Autodesk Fusion 360 part; units mm, degrees
note: some values were not read from the file. Set by a fixed rule: which sketch regions a step uses.
(part 2 of 2)
  arc A362 (-112.6, 171.1932) -> (-113.4, 170.3932) centre (-112.6, 170.3932) ccw construction
  line L338 (-117.9, 167.3932) -> (-117.9, 156.3932)
  line L339 (-117.7203, 171.6851) -> (-116.5919, 172.8135)
  line L340 (-113.9, 169.6932) -> (-113.9, 158.6932)
  line L341 (-106.1426, 173.4432) -> (-115.0716, 173.4432)
  arc A363 (-132.4, 155.6932) -> (-131.6, 154.8932) centre (-131.6, 155.6932) ccw construction
  arc A364 (-111.9, 171.6932) -> (-113.9, 169.6932) centre (-111.9, 169.6932) ccw
  line L342 (-113.4, 170.3932) -> (-113.4, 157.9932) construction
  arc A365 (-131.6, 149.8932) -> (-132.4, 149.0932) centre (-131.6, 149.0932) ccw construction
  arc A366 (-132.9, 156.3932) -> (-130.9, 154.3932) centre (-130.9, 156.3932) ccw
  line L343 (-117.6142, 171.579) -> (-116.4858, 172.7074) construction
  circle A367 centre (-115.9, 153.5432) radius 1.5
  arc A368 (-117.9, 167.3932) -> (-119.9, 169.3932) centre (-119.9, 167.3932) ccw
  line L344 (-118.4, 168.0932) -> (-118.4, 155.6932) construction
  arc A369 (-94.4, 165.9932) -> (-93.6, 165.1932) centre (-93.6, 165.9932) ccw construction
  line L345 (-92.9, 160.6932) -> (-81.9, 160.6932)
  arc A370 (-93.6, 160.1932) -> (-94.4, 159.3932) centre (-93.6, 159.3932) ccw construction
  arc A371 (-100.2, 157.1932) -> (-99.4, 157.9932) centre (-100.2, 157.9932) ccw construction
  arc A372 (-79.9, 158.6932) -> (-81.9, 160.6932) centre (-81.9, 158.6932) ccw
  arc A373 (-81.2, 165.1932) -> (-80.4, 165.9932) centre (-81.2, 165.9932) ccw construction
  arc A374 (-74.6, 163.6932) -> (-75.4, 162.8932) centre (-74.6, 162.8932) ccw construction
  arc A375 (-100.9, 156.6932) -> (-98.9, 158.6932) centre (-100.9, 158.6932) ccw
  arc A376 (-92.9, 160.6932) -> (-94.9, 158.6932) centre (-92.9, 158.6932) ccw
  arc A377 (-94.9, 166.6932) -> (-92.9, 164.6932) centre (-92.9, 166.6932) ccw
  line L346 (-93.6, 165.1932) -> (-81.2, 165.1932) construction
  arc A378 (-73.9, 164.1932) -> (-75.9, 162.1932) centre (-73.9, 162.1932) ccw
  arc A379 (-80.4, 159.3932) -> (-81.2, 160.1932) centre (-81.2, 159.3932) ccw construction
  arc A380 (-81.9, 164.6932) -> (-79.9, 166.6932) centre (-81.9, 166.6932) ccw
  line L347 (-92.9, 164.6932) -> (-81.9, 164.6932)
  arc A381 (-82.2284, 181.4432) -> (-80.9203, 181.9851) centre (-82.2284, 183.2932) ccw
  arc A382 (-73.9, 183.1932) -> (-75.9, 181.1932) centre (-73.9, 181.1932) ccw
  line L348 (-93.6, 160.1932) -> (-81.2, 160.1932) construction
  arc A383 (-82.2284, 181.2932) -> (-80.8142, 181.879) centre (-82.2284, 183.2932) ccw construction
  arc A384 (-96.0716, 181.2932) -> (-97.4858, 180.7074) centre (-96.0716, 179.2933) ccw construction
  line L349 (-96.0716, 181.2932) -> (-82.2284, 181.2932) construction
  arc A385 (-93.6, 179.1932) -> (-94.4, 178.3932) centre (-93.6, 178.3932) ccw construction
  line L350 (-77.0716, 184.9432) -> (-59.7284, 184.9432)
  arc A386 (-92.9, 179.6932) -> (-94.9, 177.6932) centre (-92.9, 177.6932) ccw
  arc A387 (-96.0716, 181.4432) -> (-97.5918, 180.8135) centre (-96.0716, 179.2933) ccw
  line L351 (-78.4858, 184.2074) -> (-80.8142, 181.879) construction
  arc A388 (-77.0716, 184.7932) -> (-78.4858, 184.2074) centre (-77.0716, 182.7933) ccw construction
  arc A389 (-75.9, 170.1932) -> (-73.9, 168.1932) centre (-73.9, 170.1932) ccw
  line L352 (-92.9, 179.6932) -> (-81.9, 179.6932)
  line L353 (-96.0716, 181.4432) -> (-82.2284, 181.4432)
  arc A390 (-79.9, 177.6932) -> (-81.9, 179.6932) centre (-81.9, 177.6932) ccw
  line L354 (-94.9, 177.6932) -> (-94.9, 166.6932)
  line L355 (-94.4, 178.3932) -> (-94.4, 165.9932) construction
  line L356 (-73.9, 164.1932) -> (-62.9, 164.1932)
  line L357 (-79.9, 177.6932) -> (-79.9, 166.6932)
  arc A391 (-77.0716, 184.9432) -> (-78.5919, 184.3135) centre (-77.0716, 182.7933) ccw
  arc A392 (-75.4, 169.4932) -> (-74.6, 168.6932) centre (-74.6, 169.4932) ccw construction
  line L358 (-75.4, 181.8932) -> (-75.4, 169.4932) construction
  line L359 (-80.4, 178.3932) -> (-80.4, 165.9932) construction
  line L360 (-73.9, 183.1932) -> (-62.9, 183.1932)
  line L361 (-78.5919, 184.3135) -> (-80.9203, 181.9851)
  line L362 (-98.9, 169.6932) -> (-98.9, 158.6932)
  arc A393 (-98.9, 169.6932) -> (-100.9, 171.6932) centre (-100.9, 169.6932) ccw
  line L363 (-75.9, 181.1932) -> (-75.9, 170.1932)
  line L364 (-93.6, 179.1932) -> (-81.2, 179.1932) construction
  arc A394 (-80.4, 178.3932) -> (-81.2, 179.1932) centre (-81.2, 178.3932) ccw construction
  arc A395 (-74.6, 182.6932) -> (-75.4, 181.8932) centre (-74.6, 181.8932) ccw construction
  arc A396 (-99.4, 170.3932) -> (-100.2, 171.1932) centre (-100.2, 170.3932) ccw construction
  line L365 (-99.4, 170.3932) -> (-99.4, 157.9932) construction
  line L366 (-73.9, 168.1932) -> (-62.9, 168.1932)
  line L367 (-80.4, 159.3932) -> (-80.4, 146.9932) construction
  line L368 (-75.4, 162.8932) -> (-75.4, 150.4932) construction
  line L369 (-74.6, 144.6932) -> (-62.2, 144.6932) construction
  circle A397 centre (-63.3, 123.4932) radius 1.5 construction
  circle A398 centre (-63.3, 123.4932) radius 3.8
  line L370 (-74.6, 130.6932) -> (-62.2, 130.6932) construction
  line L371 (-94.4, 159.3932) -> (-94.4, 146.9932) construction
  line L372 (-73.9, 149.1932) -> (-62.9, 149.1932)
  line L373 (-74.6, 182.6932) -> (-62.2, 182.6932) construction
  line L374 (-75.9, 162.1932) -> (-75.9, 151.1932)
  line L375 (-74.6, 149.6932) -> (-62.2, 149.6932) construction
  line L376 (-94.9, 158.6932) -> (-94.9, 147.6932)
  line L377 (-59.6047, 106.0356) -> (-67.8823, 120.687)
  line L378 (-74.6, 163.6932) -> (-62.2, 163.6932) construction
  line L379 (-79.9, 158.6932) -> (-79.9, 147.6932)
  line L380 (-73.9, 130.1932) -> (-62.9, 130.1932)
  line L381 (-36.6, 118.8932) -> (-24.2, 118.8932) construction
  line L382 (-36.6, 137.8932) -> (-24.2, 137.8932) construction
  line L383 (-35.9, 138.3932) -> (-24.9, 138.3932)
  line L384 (-39.0716, 102.6432) -> (-24.0284, 102.6432)
  line L385 (-36.6, 123.8932) -> (-24.2, 123.8932) construction
  circle A399 centre (-39.9, 122.5432) radius 1.5
  line L386 (-35.9, 119.3932) -> (-24.9, 119.3932)
  line L387 (-36.6, 104.8932) -> (-24.2, 104.8932) construction
  line L388 (-39.0716, 102.7932) -> (-24.0284, 102.7932) construction
  line L389 (-43.0284, 105.0932) -> (-57.7328, 105.0932) construction
  line L390 (-35.9, 123.3932) -> (-24.9, 123.3932)
  line L391 (-35.9, 104.3932) -> (-24.9, 104.3932)
  arc A400 (-37.9, 125.3932) -> (-35.9, 123.3932) centre (-35.9, 125.3932) ccw
  line L392 (-55.6, 107.1932) -> (-43.2, 107.1932) construction
  arc A401 (-41.6142, 104.5074) -> (-43.0284, 105.0932) centre (-43.0284, 103.0933) ccw construction
  arc A402 (-37.4, 105.6932) -> (-36.6, 104.8932) centre (-36.6, 105.6932) ccw construction
  line L393 (-55.6, 121.1932) -> (-43.2, 121.1932) construction
  arc A403 (-56.4, 107.9932) -> (-55.6, 107.1932) centre (-55.6, 107.9932) ccw construction
  line L394 (-40.4858, 103.379) -> (-41.6142, 104.5074) construction
  arc A404 (-59.6047, 106.0356) -> (-57.7328, 104.9432) centre (-57.7328, 107.0932) ccw
  arc A405 (-35.9, 119.3932) -> (-37.9, 117.3932) centre (-35.9, 117.3932) ccw
  line L395 (-56.9, 119.6932) -> (-56.9, 108.6932)
  arc A406 (-54.9, 121.6932) -> (-56.9, 119.6932) centre (-54.9, 119.6932) ccw
  line L396 (-56.4, 120.3932) -> (-56.4, 107.9932) construction
  arc A407 (-41.7203, 104.4013) -> (-43.0284, 104.9432) centre (-43.0284, 103.0933) ccw
  arc A408 (-41.9, 119.6932) -> (-43.9, 121.6932) centre (-43.9, 119.6932) ccw
  line L397 (-54.9, 121.6932) -> (-43.9, 121.6932)
  line L398 (-60.9, 181.1932) -> (-60.9, 170.1932)
  line L399 (-54.9, 178.6932) -> (-43.9, 178.6932)
  line L400 (-38.0797, 178.6851) -> (-39.2081, 179.8135)
  arc A409 (-42.4, 177.3932) -> (-43.2, 178.1932) centre (-43.2, 177.3932) ccw construction
  line L401 (-53.5716, 180.4432) -> (-40.7284, 180.4432)
  arc A410 (-61.4, 181.8932) -> (-62.2, 182.6932) centre (-62.2, 181.8932) ccw construction
  arc A411 (-20.7, 177.1932) -> (-21.5, 177.9932) centre (-21.5, 177.1932) ccw construction
  line L402 (-38.1858, 178.579) -> (-39.3142, 179.7074) construction
  line L403 (-36.7716, 178.1432) -> (-22.35, 178.1432)
  line L404 (-58.3142, 184.2074) -> (-54.9858, 180.879) construction
  arc A412 (-22.9, 174.3932) -> (-24.9, 176.3932) centre (-24.9, 174.3932) ccw
  arc A413 (-54.9, 178.6932) -> (-56.9, 176.6932) centre (-54.9, 176.6932) ccw
  arc A414 (-35.9, 176.3932) -> (-37.9, 174.3932) centre (-35.9, 174.3932) ccw
  arc A415 (-20.7, 176.4932) -> (-22.35, 178.1432) centre (-22.35, 176.4932) ccw
  line L405 (-36.7716, 177.9932) -> (-21.5, 177.9932) construction
  arc A416 (-39.3142, 179.7074) -> (-40.7284, 180.2932) centre (-40.7284, 178.2932) ccw construction
  arc A417 (-62.2, 168.6932) -> (-61.4, 169.4932) centre (-62.2, 169.4932) ccw construction
  arc A418 (-38.0797, 178.6851) -> (-36.7716, 178.1432) centre (-36.7716, 179.9932) ccw
  arc A419 (-60.9, 181.1932) -> (-62.9, 183.1932) centre (-62.9, 181.1932) ccw
  arc A420 (-39.2081, 179.8135) -> (-40.7284, 180.4432) centre (-40.7284, 178.2932) ccw
  arc A421 (-41.9, 176.6932) -> (-43.9, 178.6932) centre (-43.9, 176.6932) ccw
  line L406 (-53.5716, 180.2932) -> (-40.7284, 180.2932) construction
  line L407 (-36.6, 175.8932) -> (-24.2, 175.8932) construction
  line L408 (-23.4, 175.0932) -> (-23.4, 162.6932) construction
  line L409 (-37.9, 174.3932) -> (-37.9, 163.3932)
  arc A422 (-55.6, 178.1932) -> (-56.4, 177.3932) centre (-55.6, 177.3932) ccw construction
  arc A423 (-23.4, 175.0932) -> (-24.2, 175.8932) centre (-24.2, 175.0932) ccw construction
  line L410 (-35.9, 176.3932) -> (-24.9, 176.3932)
  line L411 (-58.2081, 184.3135) -> (-54.8797, 180.9851)
  arc A424 (-58.2081, 184.3135) -> (-59.7284, 184.9432) centre (-59.7284, 182.7932) ccw
  arc A425 (-38.1858, 178.579) -> (-36.7716, 177.9932) centre (-36.7716, 179.9932) ccw construction
  line L412 (-55.6, 178.1932) -> (-43.2, 178.1932) construction
  line L413 (-61.4, 181.8932) -> (-61.4, 169.4932) construction
  arc A426 (-62.9, 168.1932) -> (-60.9, 170.1932) centre (-62.9, 170.1932) ccw
  line L414 (-22.9, 174.3932) -> (-22.9, 163.3932)
  line L415 (-56.9, 176.6932) -> (-56.9, 165.6932)
  line L416 (-56.4, 177.3932) -> (-56.4, 164.9932) construction
  arc A427 (-36.6, 175.8932) -> (-37.4, 175.0932) centre (-36.6, 175.0932) ccw construction
  arc A428 (-99.4, 151.3932) -> (-100.2, 152.1932) centre (-100.2, 151.3932) ccw construction
  arc A429 (-98.9, 150.6932) -> (-100.9, 152.6932) centre (-100.9, 150.6932) ccw
  line L417 (-99.4, 151.3932) -> (-99.4, 138.9932) construction
  arc A430 (-79.9, 139.6932) -> (-81.9, 141.6932) centre (-81.9, 139.6932) ccw
  arc A431 (-93.6, 141.1932) -> (-94.4, 140.3932) centre (-93.6, 140.3932) ccw construction
  line L418 (-94.9, 139.6932) -> (-94.9, 128.6932)
  line L419 (-75.4, 143.8932) -> (-75.4, 131.4932) construction
  arc A432 (-92.9, 141.6932) -> (-94.9, 139.6932) centre (-92.9, 139.6932) ccw
  arc A433 (-100.2, 138.1932) -> (-99.4, 138.9932) centre (-100.2, 138.9932) ccw construction
  arc A434 (-81.2, 146.1932) -> (-80.4, 146.9932) centre (-81.2, 146.9932) ccw construction
  line L420 (-80.4, 140.3932) -> (-80.4, 127.9932) construction
  line L421 (-98.9, 150.6932) -> (-98.9, 139.6932)
  line L422 (-93.6, 141.1932) -> (-81.2, 141.1932) construction
  line L423 (-75.9, 143.1932) -> (-75.9, 132.1932)
  line L424 (-94.4, 140.3932) -> (-94.4, 127.9932) construction
  arc A435 (-73.9, 145.1932) -> (-75.9, 143.1932) centre (-73.9, 143.1932) ccw
  line L425 (-79.9, 139.6932) -> (-79.9, 128.6932)
  arc A436 (-100.9, 137.6932) -> (-98.9, 139.6932) centre (-100.9, 139.6932) ccw
  arc A437 (-98.1426, 114.6432) -> (-95.9152, 115.5658) centre (-98.1426, 117.7931) ccw
  line L426 (-42.4, 177.3932) -> (-42.4, 164.9932) construction
  line L427 (-61.4, 143.8932) -> (-61.4, 131.4932) construction
  line L428 (-77.0716, 184.7932) -> (-59.7284, 184.7932) construction
  line L429 (-37.4, 175.0932) -> (-37.4, 162.6932) construction
  line L430 (-20.7, 139.1932) -> (-20.7, 176.4932)
  line L431 (-60.9, 143.1932) -> (-60.9, 132.1932)
  line L432 (-41.9, 176.6932) -> (-41.9, 165.6932)
  arc A438 (-87.6574, 122.7932) -> (-89.7787, 121.9145) centre (-87.6573, 119.7931) ccw construction
  line L433 (-59.4741, 106.1094) -> (-67.7517, 120.7608) construction
  arc A439 (-100.2, 119.1932) -> (-99.4, 119.9932) centre (-100.2, 119.9932) ccw construction
  line L434 (-20.7, 139.1932) -> (-20.7, 177.1932) construction
  arc A440 (-100.9, 118.6932) -> (-98.9, 120.6932) centre (-100.9, 120.6932) ccw
  arc A441 (-94.4, 127.9932) -> (-93.6, 127.1932) centre (-93.6, 127.9932) ccw construction
  line L435 (-99.4, 132.3932) -> (-99.4, 119.9932) construction
  arc A442 (-98.1426, 114.7932) -> (-96.0213, 115.6719) centre (-98.1426, 117.7931) ccw construction
  arc A443 (-75.9, 132.1932) -> (-73.9, 130.1932) centre (-73.9, 132.1932) ccw
  line L436 (-92.9, 126.6932) -> (-81.9, 126.6932)
  line L437 (-96.0213, 115.6719) -> (-89.7787, 121.9145) construction
  line L438 (-87.6574, 122.7932) -> (-71.2344, 122.7932) construction
  arc A444 (-81.9, 126.6932) -> (-79.9, 128.6932) centre (-81.9, 128.6932) ccw
  line L439 (-95.9152, 115.5658) -> (-89.6726, 121.8084)
  arc A445 (-81.2, 127.1932) -> (-80.4, 127.9932) centre (-81.2, 127.9932) ccw construction
  arc A446 (-98.9, 131.6932) -> (-100.9, 133.6932) centre (-100.9, 131.6932) ccw
  line L440 (-93.6, 127.1932) -> (-81.2, 127.1932) construction
  arc A447 (-87.6574, 122.6432) -> (-89.6726, 121.8084) centre (-87.6573, 119.7931) ccw
  line L441 (-87.6574, 122.6432) -> (-71.2344, 122.6432)
  arc A448 (-75.4, 131.4932) -> (-74.6, 130.6932) centre (-74.6, 131.4932) ccw construction
  arc A449 (-67.7517, 120.7608) -> (-71.2344, 122.7932) centre (-71.2344, 118.793) ccw construction
  arc A450 (-67.8823, 120.687) -> (-71.2344, 122.6432) centre (-71.2344, 118.793) ccw
  line L442 (-98.9, 131.6932) -> (-98.9, 120.6932)
  arc A451 (-94.9, 128.6932) -> (-92.9, 126.6932) centre (-92.9, 128.6932) ccw
  arc A452 (-99.4, 132.3932) -> (-100.2, 133.1932) centre (-100.2, 132.3932) ccw construction
  arc A453 (-75.4, 150.4932) -> (-74.6, 149.6932) centre (-74.6, 150.4932) ccw construction
  arc A454 (-74.6, 144.6932) -> (-75.4, 143.8932) centre (-74.6, 143.8932) ccw construction
  arc A455 (-75.9, 151.1932) -> (-73.9, 149.1932) centre (-73.9, 151.1932) ccw
  line L443 (-92.9, 145.6932) -> (-81.9, 145.6932)
  arc A456 (-80.4, 140.3932) -> (-81.2, 141.1932) centre (-81.2, 140.3932) ccw construction
  arc A457 (-94.4, 146.9932) -> (-93.6, 146.1932) centre (-93.6, 146.9932) ccw construction
  arc A458 (-81.9, 145.6932) -> (-79.9, 147.6932) centre (-81.9, 147.6932) ccw
  line L444 (-93.6, 146.1932) -> (-81.2, 146.1932) construction
  arc A459 (-94.9, 147.6932) -> (-92.9, 145.6932) centre (-92.9, 147.6932) ccw
  line L445 (-92.9, 141.6932) -> (-81.9, 141.6932)
  dimension "d251" = 3.4
  dimension "d252" = 3.4
  dimension "d254" = 3.4
  dimension "d255" = 3.4
  dimension "d256" = 2
  dimension "d257" = 2
  dimension "d262" = 7.6
  dimension "d398" = 2.3
  dimension "d399" = 3
  dimension "d401" = 2.3
  dimension "d402" = 4.2
  dimension "d415" = 3
  dimension "d416" = 3
  dimension "d417" = 3
  dimension "d418" = 3
  dimension "d419" = 2
  dimension "d420" = 2
  dimension "d421" = 7.6
  dimension "d422" = 2.3
  dimension "d423" = 3
  dimension "d424" = 2.3
  dimension "d425" = 4.2
  constraint tangent L24 A23
  constraint tangent L24 A30
  constraint tangent A32 L89
  constraint tangent L41 A36
  constraint tangent L43 A98
  constraint tangent L94 A99
  constraint tangent A105 L103
  constraint tangent L98 A113
  constraint tangent L106 A112
  constraint tangent A45 L108
  constraint tangent L56 A59
  constraint tangent A62 L74
  constraint tangent A2 L65
  constraint tangent L55 A73
  constraint tangent A72 L69
  constraint tangent A5 L70
  constraint tangent L5 A53
  constraint tangent A52 L60
  constraint tangent A1 L8
  constraint tangent L0 A1
  constraint perpendicular L0 L39
  constraint perpendicular L26 L39
  constraint perpendicular L0 L10
  constraint tangent L96 A103
  constraint tangent L99 A109
  constraint tangent L102 A111
  constraint tangent A102 L104
  constraint tangent L100 A110
  constraint tangent A107 L100
  constraint tangent L31 A39
  constraint tangent L49 A46
  constraint tangent A42 L48
  constraint tangent A40 L48
  constraint tangent A43 L51
  constraint tangent A41 L46
  constraint tangent A38 L50
  constraint tangent L54 A79
  constraint tangent A57 L73
  constraint tangent A44 L53
  constraint tangent L52 A80
  constraint tangent L52 A47
  constraint tangent L34 A97
  constraint tangent L82 A91
  constraint tangent L83 A93
  constraint tangent A84 L83
  constraint tangent A84 L91
  constraint tangent L91 A104
  constraint tangent L84 A94
  constraint tangent A106 L105
  constraint tangent A100 L101
  constraint tangent A95 L95
  constraint tangent L78 A89
  constraint tangent A86 L86
  constraint tangent A92 L86
  constraint tangent L28 A77
  constraint tangent A58 L75
  constraint tangent A61 L64
  constraint tangent L76 A81
  constraint tangent L63 A81
  constraint tangent L63 A60
  constraint tangent L62 A78
  constraint tangent A82 L77
  constraint tangent L58 A82
  constraint tangent A83 L77
  constraint tangent L57 A67
  constraint tangent A14 L18
  constraint tangent A17 L42
  constraint tangent L42 A85
  constraint tangent A88 L92
  constraint tangent A37 L45
  constraint tangent A34 L44
  constraint tangent L44 A108
  constraint tangent A101 L97
  constraint tangent L32 A35
  constraint tangent A33 L40
  constraint tangent A26 L40
  constraint tangent A26 L79
  constraint tangent A20 L79
  constraint tangent A20 L22
  constraint tangent A21 L22
  constraint tangent A21 L90
  constraint tangent A24 L85
  constraint tangent A31 L85
  constraint tangent L29 A74
  constraint tangent L20 A76
  constraint tangent L17 A66
  constraint tangent L17 A68
  constraint tangent L15 A68
  constraint tangent L15 A64
  constraint tangent L19 A64
  constraint tangent L19 A15
  constraint tangent L16 A15
  constraint tangent L71 A75
  constraint tangent A69 L71
  constraint tangent L66 A69
  constraint tangent A3 L66
  constraint tangent L67 A70
  constraint tangent L7 A71
  constraint tangent L4 A12
  constraint tangent L59 A54
  constraint tangent L3 A54
  constraint tangent L3 A4
  constraint tangent A4 L7
  constraint tangent A9 L11
  constraint tangent A9 L12
  constraint tangent A0 L12
  constraint tangent A0 L14
  constraint tangent A11 L14
  constraint tangent L9 A11
  constraint tangent A8 L9
  constraint tangent A8 L11
  constraint tangent L2 A115
  constraint tangent L61 A115
  constraint tangent L2 A65
  constraint tangent A13 L72
  constraint tangent L1 A114
  constraint tangent L6 A56
  constraint tangent L38 A56
  constraint tangent L6 A63
  constraint tangent A18 L107
  constraint tangent L21 A16
  constraint tangent L25 A29
  constraint tangent L35 A29
  constraint tangent L25 A28
  constraint tangent A19 L30
  constraint tangent L23 A27
  constraint tangent A22 L26
  constraint tangent A22 L39
  constraint tangent L87 A105
  constraint tangent L80 A90
  constraint tangent L87 A96
  constraint tangent L80 A96
  constraint horizontal L10
  constraint tangent A7 L26
  constraint tangent A7 L10
  constraint tangent A10 L10
  constraint tangent L0 A10
  constraint concentric A73 A116
  constraint concentric A72 A117
  constraint concentric A5 A118
  constraint concentric A53 A119
  constraint concentric A52 A120
  constraint concentric A1 A121
  constraint concentric A23 A122
  constraint concentric A30 A123
  constraint concentric A32 A124
  constraint concentric A36 A125
  constraint concentric A98 A126
  constraint concentric A99 A127
  constraint concentric A105 A128
  constraint concentric A96 A129
  constraint concentric A90 A130
  constraint concentric A113 A131
  constraint concentric A112 A132
  constraint concentric A45 A133
  constraint concentric A59 A134
  constraint concentric A62 A135
  constraint concentric A2 A136
  constraint tangent L121 A123
  constraint tangent L115 A117
  constraint tangent A129 L128
  constraint tangent A121 L138
  constraint tangent L131 A133
  constraint tangent L128 A130
  constraint tangent A122 L121
  constraint tangent A132 L131
  constraint tangent A133 L132
  constraint tangent L132 A134
  constraint perpendicular L136 L138
  constraint coincident L137.end L138
  constraint perpendicular L137 L138
  constraint collinear L138 L139
  constraint tangent A138 L140
  constraint tangent A137 L141
  constraint tangent L111 A139
  constraint tangent L112 A139
  constraint tangent L114 A140
  constraint tangent L111 A140
  constraint tangent L112 A141
  constraint tangent L113 A141
  constraint tangent L114 A142
  constraint tangent L113 A142
  constraint tangent A145 L145
  constraint tangent L144 A145
  constraint tangent A146 L146
  constraint tangent L145 A146
  constraint tangent A144 L144
  constraint tangent L143 A144
  constraint tangent A143 L146
  constraint tangent A143 L143
  constraint tangent L148 A148
  constraint tangent A148 L149
  constraint tangent L147 A147
  constraint tangent A147 L148
  constraint tangent L149 A149
  constraint tangent A149 L150
  constraint tangent L147 A150
  constraint tangent L150 A150
  constraint tangent L152 A152
  constraint tangent A152 L153
  constraint tangent L151 A151
  constraint tangent A151 L152
  constraint tangent L153 A153
  constraint tangent A153 L154
  constraint tangent L151 A154
  constraint tangent L154 A154
  constraint tangent L156 A156
  constraint tangent A156 L157
  constraint tangent L155 A155
  constraint tangent A155 L156
  constraint tangent L157 A157
  constraint tangent A157 L158
  constraint tangent L155 A158
  constraint tangent L158 A158
  constraint tangent L160 A160
  constraint tangent A160 L161
  constraint tangent L159 A159
  constraint tangent A159 L160
  constraint tangent L161 A161
  constraint tangent A161 L162
  constraint tangent L159 A162
  constraint tangent L162 A162
  constraint tangent L164 A164
  constraint tangent A164 L165
  constraint tangent L163 A163
  constraint tangent A163 L164
  constraint tangent L165 A165
  constraint tangent A165 L166
  constraint tangent L163 A166
  constraint tangent L166 A166
  constraint tangent L168 A168
  constraint tangent A168 L169
  constraint tangent L167 A167
  constraint tangent A167 L168
  constraint tangent L169 A169
  constraint tangent A169 L170
  constraint tangent L167 A170
  constraint tangent A170 L170
  constraint tangent L172 A172
  constraint tangent A172 L173
  constraint tangent L171 A171
  constraint tangent A171 L172
  constraint tangent L173 A173
  constraint tangent A173 L174
  constraint tangent L171 A174
  constraint tangent A174 L174
  constraint tangent L176 A176
  constraint tangent A176 L177
  constraint tangent L175 A175
  constraint tangent A175 L176
  constraint tangent L177 A177
  constraint tangent A177 L178
  constraint tangent L175 A178
  constraint tangent A178 L178
  constraint tangent L180 A180
  constraint tangent A180 L181
  constraint tangent L179 A179
  constraint tangent A179 L180
  constraint tangent L181 A181
  constraint tangent A181 L182
  constraint tangent L179 A182
  constraint tangent A182 L182
  constraint tangent L184 A184
  constraint tangent A184 L185
  constraint tangent L183 A183
  constraint tangent A183 L184
  constraint tangent L185 A185
  constraint tangent A185 L186
  constraint tangent L183 A186
  constraint tangent A186 L186
  constraint tangent L192 A192
  constraint tangent A192 L193
  constraint tangent L191 A191
  constraint tangent A191 L192
  constraint tangent L193 A193
  constraint tangent A193 L194
  constraint tangent L191 A194
  constraint tangent A194 L194
  constraint tangent L188 A188
  constraint tangent A188 L189
  constraint tangent L187 A187
  constraint tangent A187 L188
  constraint tangent L189 A189
  constraint tangent A189 L190
  constraint tangent L187 A190
  constraint tangent L190 A190
  constraint tangent L196 A196
  constraint tangent A196 L197
  constraint tangent L195 A195
  constraint tangent A195 L196
  constraint tangent L197 A197
  constraint tangent A197 L198
  constraint tangent L195 A198
  constraint tangent A198 L198
  constraint tangent L200 A200
  constraint tangent A200 L201
  constraint tangent L199 A199
  constraint tangent A199 L200
  constraint tangent L201 A201
  constraint tangent A201 L202
  constraint tangent L199 A202
  constraint tangent A202 L202
  constraint tangent L204 A204
  constraint tangent A204 L205
  constraint tangent L203 A203
  constraint tangent A203 L204
  constraint tangent L205 A205
  constraint tangent A205 L206
  constraint tangent L203 A206
  constraint tangent A206 L206
  constraint tangent L208 A208
  constraint tangent A208 L209
  constraint tangent L207 A207
  constraint tangent A207 L208
  constraint tangent L209 A209
  constraint tangent A209 L210
  constraint tangent L207 A210
  constraint tangent A210 L210
  constraint tangent L212 A212
  constraint tangent A212 L213
  constraint tangent L211 A211
  constraint tangent A211 L212
  constraint tangent L213 A213
  constraint tangent A213 L214
  constraint tangent L211 A214
  constraint tangent L214 A214
  constraint tangent L216 A216
  constraint tangent A216 L217
  constraint tangent L215 A215
  constraint tangent A215 L216
  constraint tangent L217 A217
  constraint tangent A217 L218
  constraint tangent L215 A218
  constraint tangent A218 L218
  constraint tangent L220 A219
  constraint tangent A219 L221
  constraint tangent L221 A220
  constraint tangent A220 L222
  constraint tangent L220 A221
  constraint tangent L219 A221
  constraint tangent L219 A222
  constraint tangent L222 A222
  constraint concentric A49 A224
  constraint concentric A225 A226
  constraint tangent L120 A227
  constraint tangent L27 A227
  constraint coincident L0 A55.end
  constraint tangent L139 A228
  constraint tangent L142 A228
  constraint tangent L110 A229
  constraint tangent L142 A229
  constraint tangent L402 A425
  constraint tangent L402 A416
  constraint tangent A298 L406
  constraint tangent A301 L404
  constraint tangent A388 L428
  constraint tangent A383 L351
  constraint tangent A384 L349
  constraint tangent A352 L343
  constraint tangent A327 L336
  constraint tangent A332 L327
  constraint tangent L301 A442
  constraint tangent A438 L437
  constraint tangent L438 A449
  constraint tangent A246 L433
  constraint tangent L389 A401
  constraint tangent A244 L394
  constraint tangent A272 L388
  constraint tangent L249 A265
  constraint tangent L248 A281
  constraint tangent L253 A281
  constraint perpendicular L253 L405
  constraint perpendicular L405 L434
  constraint perpendicular L237 L253
  constraint tangent L297 A328
  constraint tangent L295 A356
  constraint tangent A359 L344
  constraint tangent L292 A363
  constraint tangent L296 A365
  constraint tangent L296 A350
  constraint tangent A348 L334
  constraint tangent L321 A346
  constraint tangent L306 A345
  constraint tangent L306 A335
  constraint tangent A343 L330
  constraint tangent A331 L333
  constraint tangent L298 A344
  constraint tangent L310 A439
  constraint tangent L435 A452
  constraint tangent L305 A336
  constraint tangent L308 A433
  constraint tangent L308 A355
  constraint tangent A326 L324
  constraint tangent L311 A428
  constraint tangent A325 L314
  constraint tangent L314 A371
  constraint tangent A371 L365
  constraint tangent A396 L365
  constraint tangent L302 A362
  constraint tangent A385 L355
  constraint tangent L364 A394
  constraint tangent A373 L359
  constraint tangent A369 L346
  constraint tangent A370 L348
  constraint tangent A379 L348
  constraint tangent L367 A434
  constraint tangent A457 L444
  constraint tangent A431 L422
  constraint tangent L424 A441
  constraint tangent A441 L440
  constraint tangent A445 L440
  constraint tangent L420 A456
  constraint tangent L419 A448
  constraint tangent L370 A448
  constraint tangent L419 A454
  constraint tangent A293 L369
  constraint tangent A283 L427
  constraint tangent A290 L375
  constraint tangent L375 A453
  constraint tangent A374 L368
  constraint tangent A292 L378
  constraint tangent L307 A417
  constraint tangent L307 A392
  constraint tangent L358 A395
  constraint tangent L373 A410
  constraint tangent A422 L416
  constraint tangent A295 L416
  constraint tangent A295 L272
  constraint tangent A288 L272
  constraint tangent A288 L426
  constraint tangent A409 L426
  constraint tangent A409 L412
  constraint tangent L269 A303
  constraint tangent L269 A297
  constraint tangent L271 A299
  constraint tangent L270 A317
  constraint tangent L230 A282
  constraint tangent A236 L230
  constraint tangent A236 L226
  constraint tangent L226 A239
  constraint tangent A239 L228
  constraint tangent L228 A241
  constraint tangent A241 L265
  constraint tangent A232 L393
  constraint tangent A245 L393
  constraint tangent A245 L396
  constraint tangent A403 L396
  constraint tangent A231 L392
  constraint tangent L232 A402
  constraint tangent A262 L387
  constraint tangent L254 A269
  constraint tangent A269 L381
  constraint tangent A230 L381
  constraint tangent A230 L232
  constraint tangent A271 L257
  constraint tangent L252 A271
  constraint tangent L252 A276
  constraint tangent L263 A276
  constraint tangent L263 A275
  constraint tangent L247 A275
  constraint tangent L247 A268
  constraint tangent A268 L257
  constraint tangent A248 L385
  constraint tangent A248 L238
  constraint tangent A238 L385
  constraint tangent L264 A285
  constraint tangent A252 L382
  constraint tangent A308 L281
  constraint tangent L278 A308
  constraint tangent A310 L281
  constraint tangent L283 A319
  constraint tangent L276 A312
  constraint tangent A307 L280
  constraint tangent A307 L408
  constraint tangent L280 A318
  constraint tangent A427 L429
  constraint tangent L407 A423
  constraint tangent A411 L434
  constraint tangent A411 L405
  constraint tangent L312 A384
  constraint tangent L294 A358
  constraint tangent A321 L312
  constraint tangent A321 L294
  constraint horizontal L237
  constraint tangent A259 L434
  constraint tangent L237 A259
  constraint tangent L237 A256
  constraint tangent A256 L253
  constraint concentric A246 A404
  constraint concentric A401 A407
  constraint concentric A244 A247
  constraint concentric A272 A273
  constraint concentric A265 A270
  constraint concentric A277 A281
  constraint concentric A418 A425
  constraint concentric A416 A420
  constraint concentric A298 A302
  constraint concentric A301 A424
  constraint concentric A388 A391
  constraint concentric A381 A383
  constraint concentric A384 A387
  constraint concentric A321 A361
  constraint concentric A351 A358
  constraint concentric A352 A353
  constraint concentric A322 A327
  constraint concentric A332 A347
  constraint concentric A437 A442
  constraint concentric A438 A447
  constraint concentric A449 A450
  constraint tangent L400 A420
  constraint tangent L223 A407
  constraint tangent A361 L341
  constraint tangent L256 A277
  constraint tangent A347 L325
  constraint tangent A351 L341
  constraint tangent L400 A418
  constraint tangent A322 L325
  constraint tangent L319 A347
  constraint tangent L319 A437
  constraint perpendicular L256 L261
  constraint coincident L259.start L256
  constraint perpendicular L256 L260
  constraint collinear L256 L259
  constraint tangent L239 A266
  constraint tangent A263 L262
  constraint tangent L289 A324
  constraint tangent L293 A324
  constraint tangent L338 A368
  constraint tangent L289 A368
  constraint tangent L293 A366
  constraint tangent L337 A366
  constraint tangent A338 L338
  constraint tangent A338 L337
  constraint tangent L303 A364
  constraint tangent L340 A364
  constraint tangent L362 A393
  constraint tangent L303 A393
  constraint tangent A339 L340
  constraint tangent L320 A339
  constraint tangent A375 L362
  constraint tangent L320 A375
  constraint tangent A386 L352
  constraint tangent A386 L354
  constraint tangent A390 L357
  constraint tangent L352 A390
  constraint tangent A377 L354
  constraint tangent A377 L347
  constraint tangent A380 L357
  constraint tangent A380 L347
  constraint tangent A382 L360
  constraint tangent A382 L363
  constraint tangent L398 A419
  constraint tangent L360 A419
  constraint tangent A389 L363
  constraint tangent A389 L366
  constraint tangent L398 A426
  constraint tangent L366 A426
  constraint tangent L399 A413
  constraint tangent A413 L415
  constraint tangent A421 L432
  constraint tangent L399 A421
  constraint tangent A294 L415
  constraint tangent A294 L287
  constraint tangent A316 L432
  constraint tangent A316 L287
  constraint tangent A414 L410
  constraint tangent A414 L409
  constraint tangent A412 L414
  constraint tangent A412 L410
  constraint tangent A311 L409
  constraint tangent A311 L282
  constraint tangent A304 L414
  constraint tangent A304 L282
  constraint tangent L291 A323
  constraint tangent A323 L322
  constraint tangent L329 A357
  constraint tangent L291 A357
  constraint tangent A334 L322
  constraint tangent L304 A334
  constraint tangent A340 L329
  constraint tangent L304 A340
  constraint tangent L317 A360
  constraint tangent L326 A360
  constraint tangent A429 L421
  constraint tangent L317 A429
  constraint tangent A329 L326
  constraint tangent A329 L313
  constraint tangent L421 A436
  constraint tangent L313 A436
  constraint tangent L345 A376
  constraint tangent A376 L376
  constraint tangent A372 L379
  constraint tangent L345 A372
  constraint tangent L376 A459
  constraint tangent L443 A459
  constraint tangent L379 A458
  constraint tangent L443 A458
  constraint tangent A378 L356
  constraint tangent A378 L374
  constraint tangent A291 L284
  constraint tangent A291 L356
  constraint tangent L374 A455
  constraint tangent L372 A455
  constraint tangent A296 L284
  constraint tangent A296 L372
  constraint tangent A315 L288
  constraint tangent L268 A315
  constraint tangent A287 L274
  constraint tangent A287 L288
  constraint tangent L268 A300
  constraint tangent L273 A300
  constraint tangent A289 L274
  constraint tangent A289 L273
  constraint tangent A305 L279
  constraint tangent L275 A305
  constraint tangent A313 L286
  constraint tangent L279 A313
  constraint tangent L275 A306
  constraint tangent L277 A306
  constraint tangent L286 A320
  constraint tangent L277 A320
  constraint tangent L299 A354
  constraint tangent L323 A354
  constraint tangent L309 A337
  constraint tangent L299 A337
  constraint tangent A330 L323
  constraint tangent A330 L331
  constraint tangent A333 L309
  constraint tangent A333 L331
  constraint tangent L300 A349
  constraint tangent A349 L335
  constraint tangent A446 L442
  constraint tangent L300 A446
  constraint tangent A342 L335
  constraint tangent L316 A342
  constraint tangent A440 L442
  constraint tangent L316 A440
  constraint tangent A432 L445
  constraint tangent L418 A432
  constraint tangent A430 L425
  constraint tangent A430 L445
  constraint tangent L418 A451
  constraint tangent L436 A451
  constraint tangent L425 A444
  constraint tangent L436 A444
  constraint tangent L318 A435
  constraint tangent L423 A435
  constraint tangent A314 L431
  constraint tangent A314 L318
  constraint tangent L423 A443
  constraint tangent L380 A443
  constraint tangent A286 L431
  constraint tangent A286 L380
  constraint tangent A242 L231
  constraint tangent L225 A242
  constraint tangent A284 L266
  constraint tangent L231 A284
  constraint tangent A237 L225
  constraint tangent A237 L227
  constraint tangent A235 L266
  constraint tangent A235 L227
  constraint tangent A240 L383
  constraint tangent A240 L229
  constraint tangent L240 A258
  constraint tangent A258 L383
  constraint tangent L229 A400
  constraint tangent L390 A400
  constraint tangent A254 L240
  constraint tangent A254 L390
  constraint tangent A406 L397
  constraint tangent L395 A406
  constraint tangent L224 A408
  constraint tangent A408 L397
  constraint tangent A233 L395
  constraint tangent A233 L235
  constraint tangent L224 A243
  constraint tangent A243 L235
  constraint tangent L386 A405
  constraint tangent L234 A405
  constraint tangent L243 A264
  constraint tangent A264 L386
  constraint tangent A234 L234
  constraint tangent A234 L391
  constraint tangent L243 A274
  constraint tangent A274 L391
  constraint tangent L250 A267
  constraint tangent L242 A267
  constraint tangent L242 A261
  constraint tangent A261 L246
  constraint tangent L250 A278
  constraint tangent L255 A278
  constraint tangent L255 A280
  constraint tangent L246 A280
  constraint concentric A397 A398
  constraint concentric A249 A253
  constraint tangent L403 A415
  constraint tangent A415 L430
  constraint coincident A251.end L253
  constraint tangent L259 A279
  constraint tangent L245 A279
  constraint tangent L241 A260
  constraint tangent A260 L245
  measures "d251" diameter of A87
  measures "d252" diameter of A48
  measures "d254" diameter of A6
  measures "d255" diameter of A25
  measures "d256" diameter of A50
  measures "d257" diameter of A51
  measures "d262" diameter of A49
  measures "d398" diameter of A223
  measures "d399" diameter of A224
  measures "d401" diameter of A225
  measures "d402" diameter of A226
  measures "d415" diameter of A367
  measures "d416" diameter of A341
  measures "d417" diameter of A399
  measures "d418" diameter of A309
  measures "d419" diameter of A255
  measures "d420" diameter of A257
  measures "d421" diameter of A398
  measures "d422" diameter of A250
  measures "d423" diameter of A397
  measures "d424" diameter of A249
  measures "d425" diameter of A253
extrude "Extrude19" add sketch "mriya-spacer-fdm" along normal blind 3.4 contours L13 L27 L110 A116 L115 A117 L116 A118 L117 A119 L118 A120 L119 A121 L120 A122 L121 A123 L122 A124 L123 A125 L124 A126 L125 A127 L126 A128 L127 A129 L128 A130 L129 A131 L130 A132 L131 A133 L132 A134 L133 A135 L134 A136 L135 L136 L137 L138 L139 L142 A227 A228 A229 makes body 1
fillet "Fillet10" radius 0.8 2 edges at (-2.8, 5.0932, 1.7) (-2.8, 14.0932, 1.7) on bodies 1
fillet "Fillet11" radius 0.6 2 edges at (-1.95, 5.0932, 1.7) (-1.95, 14.0932, 1.7) on bodies 1
mirror "Mirror5" about plane through (0, 0, 0) normal (1, 0, 0) of bodies 1 makes body 2
extrude "Extrude28" add sketch "mriya-spacer-fdm" along normal blind 3.4 separate body contours L223 L236 A247 L241 A260 L244 L245 L251 A270 L256 L258 A273 L259 L260 L261 A277 A279 A302 L290 A322 L315 L319 A347 L325 A351 A353 A361 L339 L341 A381 L350 A387 L353 A391 L361 L377 L384 A404 A407 L400 L401 L403 A415 A418 A420 L411 A424 A437 L430 L439 A447 L441 A450 makes body 3
fillet "Fillet14" radius 0.8 2 edges at (-2.8, 114.0932, 1.7) (-2.8, 105.0932, 1.7) on bodies 3
fillet "Fillet15" radius 0.6 2 edges at (-1.95, 114.0932, 1.7) (-1.95, 105.0932, 1.7) on bodies 3
mirror "Mirror8" about plane through (0, 0, 0) normal (1, 0, 0) of bodies 3 makes body 4
named bodies: "right", "left", "right-inserts", "left-inserts"
